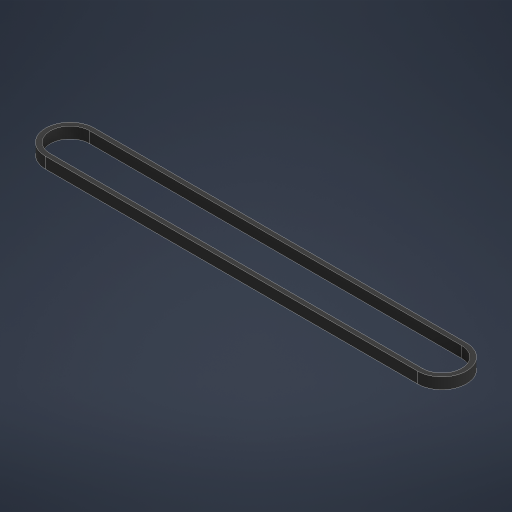
# Autodesk Inventor part: CORL_012_ArmBelt
Saved by Autodesk Inventor 2024.2 (Build 282272000, 272)
## iProperties
Created: 2024-08-05
Part Number: CORL_012_ArmBelt
Material: Rubber, Silicone
Document SubType Name: Modeling
Designer: Bryan
Density: 1.25 g/cm^3
Appearance: Rubber - Black
Mass: 22.6322 g
Surface Area: 182.8 cm^2
Volume: 18.1058 cm^3
Author: Bryan
Autodesk Inventor part; units mm, degrees
ref_plane "YZ Plane" through (0, 0, 0) normal (1, 0, 0) x (0, 1, 0)
ref_plane "XZ Plane" through (0, 0, 0) normal (0, 1, 0) x (-1, 0, 0)
ref_plane "XY Plane" through (0, 0, 0) normal (0, 0, 1) x (1, 0, 0)
sketch "Sketch1" plane through (0, 0, 0) normal (0, 1, 0) x (-1, 0, 0)
  line L0 (0, 0) -> (299.9994, 0) construction
  line L1 (299.9994, 19.7231) -> (0, 19.7231)
  arc A0 (299.9994, -19.7231) -> (299.9994, 19.7231) centre (299.9994, 0) ccw
  arc A1 (0, 19.7231) -> (0, -19.7231) centre (0, 0) ccw
  line L2 (0, 15.9131) -> (299.9994, 15.9131)
  arc A2 (299.9994, -15.9131) -> (299.9994, 15.9131) centre (299.9994, 0) ccw
  line L3 (299.9994, -15.9131) -> (0, -15.9131)
  arc A3 (0, 15.9131) -> (0, -15.9131) centre (0, 0) ccw
  circle A4 centre (0, 0) radius 15.9131 construction
  line L4 (299.9994, -19.7231) -> (0, -19.7231)
  dimension "d8" = 31.8262
  dimension "d1" = 299.9994
  dimension "d7" = 3.81
  constraints: 10 end point, 8 point on circle, 6 horizontal, 4 centre point, 4 coincident, 3 tangent, 1 equal radius, 1 vertical alignment, 3 other
  measures "d1" distance of L0.start L0.end
  measures "d7" distance between parallel lines of L1 L2
extrude "Extrusion1" add sketch "Sketch1" along normal blind 9
body "Solid1"
